Ring v4 (Autodesk Fusion 360 design; units mm, degrees)
Autodesk Fusion 360 part; units mm, degrees
sketch "Sketch1" plane through (0, 0, 0) normal (0, 1, 0) x (1, 0, 0)
  circle A0 centre (0, 0) radius 25.4 construction
  circle A1 centre (0, 0) radius 24.65
  circle A2 centre (0, 0) radius 20.65
  dimension "d6" = -0.75
  dimension "d7" = 50.8
  dimension "d8" = -4.75
  constraint coincident A0.centre A1.centre
  measures "d7" diameter of A0
extrude "Extrude1" add sketch "Sketch1" along normal mid plane 20
sketch "Sketch3" plane through (0, -10, 0) normal (0, -1, 0) x (1, 0, 0)
  circle A0 centre (0, 0) radius 20.65
  line L0 (0, 0) -> (20.65, 0) construction
  circle A1 centre (13.15, 0) radius 7.5
  circle A2 centre (13.15, 0) radius 5.5
  line L1 (19.2399, -7.5) -> (-1.0882, -7.5) construction
  arc A3 (15.837, -13.2519) -> (13.15, -7.5) centre (13.15, -11.0035) ccw
  arc A4 (13.15, 7.5) -> (15.837, 13.2519) centre (13.15, 11.0035) ccw
  circle A5 centre (0, 0) radius 20.65
  circle A6 centre (0, 0) radius 24.65
  dimension "d9" = 15
  dimension "d10" = -2
  constraint coincident A0.centre L0.start
  constraint coincident A0 L0.end
  constraint horizontal L0
  constraint coincident L0.end A1
  constraint tangent A0 A1
  constraint coincident A0 L1.start
  constraint parallel L0 L1
  constraint tangent A1 L1
  constraint coincident A0 A3.start
  constraint coincident A1 A3.end
  constraint tangent A1 A3
  constraint tangent A0 A3
  constraint coincident L1 A3.end
  constraint symmetric L0 A3.end A4.start
  constraint symmetric L0 A3.start A4.end
  constraint symmetric L0 A3 A4
  measures "d9" diameter of A1
extrude "Extrude2" add sketch "Sketch3" against normal blind 4 contours A0 A1 A4 A5 | A1 | A0 A1 A3 A5
fillet "Fillet3" radius 1 2 edges at (8.0222, -6, -1.9889) (8.0222, -10, 1.9889)
fillet "Fillet4" radius 0.5 2 edges at (16.3243, -6, -9.5207) (5.65, -6, 0.0045)
fillet "Fillet4" radius 0.5 1 edges at (16.3262, -6, 9.5248)
equation "cardboard_offset = -0.75 mm"
equation "d6 = cardboard_offset"
equation "d8 = cardboard_offset - 4 mm"
